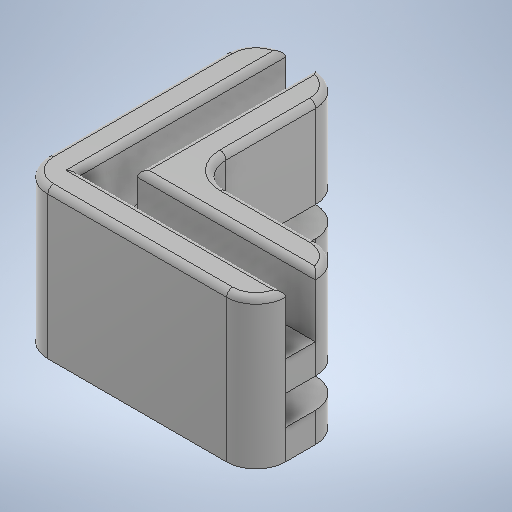
# Autodesk Inventor part: TSU_Corner1_Clamp
Saved by Autodesk Inventor 2025.2 (Build 292293000, 293)
## iProperties
Created: 2025-01-07
Part Number: TSU_Corner1_Clamp
Material: Generic
Document SubType Name: Modeling
Designer: Matt Tidd
Density: 1 g/cm^3
Appearance: Default
Author: Matt Tidd
Autodesk Inventor part; units mm, degrees
ref_plane "YZ Plane" through (0, 0, 0) normal (1, 0, 0) x (0, 1, 0)
ref_plane "XZ Plane" through (0, 0, 0) normal (0, 1, 0) x (-1, 0, 0)
ref_plane "XY Plane" through (0, 0, 0) normal (0, 0, 1) x (1, 0, 0)
sketch "Sketch1" plane through (0, 0, 0) normal (0, 1, 0) x (-1, 0, 0)
  line L0 (0, 0) -> (145, 0)
  line L1 (145, 0) -> (145, -30)
  line L2 (145, -30) -> (0, -30)
  line L3 (0, -30) -> (0, 0)
  line L4 (145, 0) -> (115, 0)
  line L5 (115, 0) -> (115, -70)
  line L6 (115, -70) -> (145, -70)
  line L7 (145, -70) -> (145, 0)
  point P0 (115, -30)
  dimension "d0" = 145
  dimension "d1" = 30
  dimension "d2" = 30
  dimension "d3" = 70
  constraints: 16 end point, 4 parallel, 2 horizontal, 2 perpendicular
  measures "d0" distance of L1.end L2.end
  measures "d1" distance of L0.end L1.end
  measures "d2" distance of L6.end L5.end
  measures "d3" distance of L5.end L4.end
extrude "Extrusion1" add sketch "Sketch1" along normal blind 30
sketch "Sketch2" plane through (0, 0, -30) normal (0, 0, -1) x (-1, 0, 0)
  line L0 (0, 20) -> (135, 20)
  line L1 (135, 20) -> (135, 10)
  line L2 (135, 10) -> (0, 10)
  line L3 (0, 10) -> (0, 20)
  dimension "d32" = 135
  dimension "d33" = 10
  constraints: 8 end point, 2 parallel, 1 horizontal, 1 perpendicular
  measures "d32" distance of L1.end L2.end
  measures "d33" distance of L0.end L1.end
extrude "Extrusion2" cut sketch "Sketch2" along normal blind 50 and the other way blind 20
sketch "Sketch4" plane through (0, 30, 0) normal (0, 1, 0) x (1, 0, 0)
  line L0 (0, 0) -> (-145, 0)
  line L1 (-145, 0) -> (-145, 10)
  line L2 (-145, 10) -> (0, 10)
  line L3 (0, 10) -> (0, 0)
  line L4 (-115, 70) -> (-145, 70) projected
  line L5 (-145, 70) -> (-135, 70)
  line L6 (-135, 70) -> (-135, 10)
  line L7 (-135, 10) -> (-145, 10)
  line L8 (-145, 10) -> (-145, 70)
  line L9 (-115, 30) -> (-115, 70) projected
  line L10 (-115, 70) -> (-125, 70)
  line L11 (-125, 70) -> (-125, 30)
  line L12 (-125, 30) -> (-115, 30)
  line L13 (-115, 30) -> (-115, 70)
  line L14 (0, 30) -> (-125, 30)
  line L15 (-125, 30) -> (-125, 20)
  line L16 (-125, 20) -> (0, 20)
  line L17 (0, 20) -> (0, 30)
  dimension "d22" = 145
  dimension "d23" = 10
  dimension "d24" = 10
  dimension "d25" = 60
  dimension "d26" = 10
  dimension "d27" = 40
  dimension "d28" = 125
  dimension "d29" = 10
  constraints: 32 end point, 8 parallel, 4 horizontal, 4 perpendicular, 2 point on line
  measures "d22" distance of L1.end L2.end
  measures "d23" distance of L0.end L1.end
  measures "d24" distance of L6.end L7.end
  measures "d25" distance of L5.end L6.end
  measures "d26" distance of L12.end L11.end
  measures "d27" distance of L11.end L10.end
  measures "d28" distance of L16.end L15.end
  measures "d29" distance of L15.end L14.end
extrude "Extrusion4" add sketch "Sketch4" along normal blind 20
sketch "Sketch5" plane through (0, 0, 0) normal (1, 0, 0) x (0, 0, -1)
  line L0 (0, 0) -> (0, 50) projected
  line L1 (30, 0) -> (30, 10) projected
  line L2 (0, 50) -> (30, 50)
  line L3 (30, 50) -> (30, 0)
  line L4 (30, 0) -> (0, 0)
  line L5 (0, 0) -> (0, 50)
  constraints: 8 end point, 2 parallel, 1 horizontal, 1 perpendicular
extrude "Extrusion5" cut sketch "Sketch5" against normal blind 65
sketch "Sketch6" plane through (-115, 0, -70) normal (0, 0, -1) x (-1, 0, 0)
  line L0 (20, 10) -> (0, 10) projected
  line L1 (0, 0) -> (0, 10) projected
  line L2 (0, 0) -> (30, 0) projected
  line L3 (30, 0) -> (30, 50) projected
  line L4 (20, 50) -> (30, 50) projected
  line L5 (20, 30) -> (20, 50) projected
  line L6 (10, 30) -> (20, 30) projected
  line L7 (10, 30) -> (10, 50) projected
  line L8 (0, 50) -> (10, 50) projected
  line L9 (0, 20) -> (0, 50) projected
  line L10 (0, 20) -> (20, 20) projected
  line L11 (20, 20) -> (20, 10) projected
  point P0 (-115, 0)
extrude "Extrusion6" add sketch "Sketch6" along normal blind 10
fillet "Fillet1" radius 9.9 9 edges at (-115, 35, -30) (-115, 5, -30) (-115, 35, -80) (-115, 5, -80) (-65, 35, -30) (-65, 5, -30) (-145, 25, -80) (-65, 25, 0) (-145, 25, 0)
fillet "Fillet2" radius 2 18 edges at (-67.8996, 50, -2.8996) (-65, 50, -9.95) (-142.1004, 50, -2.8996) (-145, 50, -40) (-142.1004, 50, -77.1004) (-135.05, 50, -80) (-105, 50, 0) (-100, 50, -10) (-125, 50, -50) (-95, 50, -20) (-112.1004, 50, -32.8996) (-115, 50, -55) (-117.8996, 50, -77.1004) (-124.95, 50, -80) (-67.8996, 50, -27.1004) (-65, 50, -20.05) (-90, 50, -30) (-135, 50, -45)
body "Solid1"
